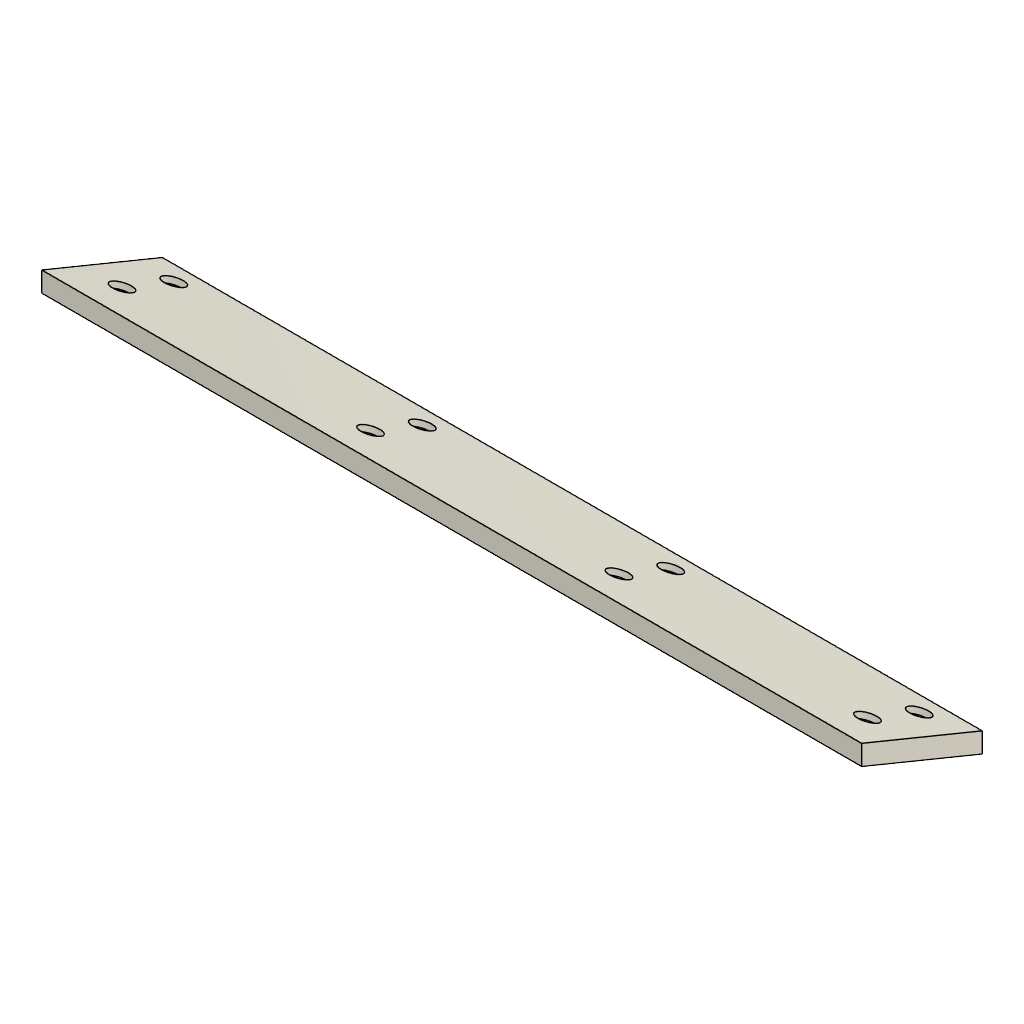
name_sign_LED_holder_bottom (Autodesk Fusion 360 design; units mm, degrees)
part number: 2026-10-25-14-42-28-917
Autodesk Fusion 360 part; units mm, degrees
sketch "Name sign LED holder bottom" plane through (0, 0, 0) normal (1, 0, 0) x (0, 1, 0)
  line L0 (0, 18.6852) -> (0, 13.281)
  line L1 (0, 13.281) -> (32.3823, 0)
  line L2 (32.3823, 0) -> (32.3823, 5.4042)
  line L3 (32.3823, 5.4042) -> (0, 18.6852)
  point P0 (0, 13.281)
  dimension "d1" = 5
  dimension "d2" = 112.3
  dimension "d3" = 35
  dimension "d4" = 5.4042
  dimension "d5" = 5.4042
  constraint vertical L0
  constraint parallel L1 L3
  constraint parallel L0 L2
  constraint coincident P0 L0.end
  measures "d1" distance of L1 L3
  measures "d2" angle of L0 L3
  measures "d3" distance of P0 L1.end
  measures "d4" distance of L0.start P0
  measures "d5" distance of L1.end L2.end
extrude "Extrude1" add sketch "Name sign LED holder bottom" along normal blind 220
sketch "Magnet holes" plane through (0, 6.5599, 15.9948) normal (0, 0.379456, 0.92521) x (-1, 0, 0)
  line L0 (0, -27.9098) -> (0, 7.0902)
  line L1 (0, 7.0902) -> (-220, 7.0902)
  line L2 (-220, 7.0902) -> (-220, -27.9098)
  line L3 (-220, -27.9098) -> (0, -27.9098)
  circle A0 centre (-210, -20.4098) radius 2.75
  dimension "d17" = 5.5
  dimension "d18" = 10
  dimension "d19" = 7.5
  measures "d17" diameter of A0
  measures "d18" distance of L2 A0.centre
  measures "d19" distance of L3 A0.centre
extrude "Extrude2" cut sketch "Magnet holes" against normal blind 1.5 contours A0
pattern_linear "R-Pattern1" count 4 spacing 66.6667 along (-1, 0, 0) count 2 spacing 15 along (0, -0.92521, 0.379456) of "Extrude2"
equation "magnet_hole_diameter = 5.5 mm"
equation "magnet_hole_depth = 1.5 mm"
equation "number_of_magnet_columns = 4"
equation "number_of_magnet_rows = 2"
equation "magnet_hole_side_offset = 10 mm"
equation "magnet_hole_top_offset = 7.5 mm"
equation "magnet_pattern_length = 220.00 mm - 2 * ( magnet_hole_side_offset )"
equation "d17 = magnet_hole_diameter"
equation "d18 = magnet_hole_side_offset"
equation "d19 = magnet_hole_top_offset"
equation "d20 = -magnet_hole_depth"
equation "d22 = number_of_magnet_columns"
equation "d23 = number_of_magnet_rows"
equation "d24 = magnet_pattern_length"
equation "d25 = magnet_pattern_height"
equation "vertical_part_width = 5.00 mm"
equation "magnet_pattern_height = 35.00 mm - vertical_part_width - 2 * ( magnet_hole_top_offset )"
named bodies: "Name sign LED holder bottom"
